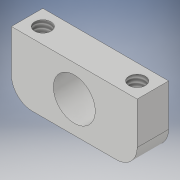
# Autodesk Inventor part: WheelSuspensionHub
Saved by Autodesk Inventor 2017 (Build 210142000, 142)
## iProperties
Created: 2018-05-04
Part Number: WheelSuspensionHub
Material: Generic
Document SubType Name: Modeling
Designer: User
Density: 1 g/cm^3
Appearance: Default
Author: User
Autodesk Inventor part; units mm, degrees
ref_plane "YZ Plane" through (0, 0, 0) normal (1, 0, 0) x (0, 1, 0)
ref_plane "XZ Plane" through (0, 0, 0) normal (0, 1, 0) x (-1, 0, 0)
ref_plane "XY Plane" through (0, 0, 0) normal (0, 0, 1) x (1, 0, 0)
sketch "Sketch1" plane through (0, 0, 0) normal (0, 0, 1) x (1, 0, 0)
  circle A0 centre (0, 0) radius 6.35
  arc A1 (0, 9.525) -> (0, -9.525) centre (0, 0) ccw
  line L0 (0, -9.525) -> (19.05, -9.525)
  line L1 (19.05, -9.525) -> (19.05, 9.525)
  line L2 (19.05, 9.525) -> (0, 9.525)
  dimension "d0" = 12.7
  dimension "d1" = 19.05
  dimension "d2" = 19.05
  dimension "d3" = 19.05
  constraints: 6 end point, 2 centre point, 2 coincident, 2 point on circle, 2 tangent, 1 horizontal, 1 vertical
  measures "d0" diameter of A0
  measures "d1" diameter of A1
  measures "d2" distance of L0.start L0.end
  measures "d3" distance of L0.end L1.end
extrude "Extrusion1" add sketch "Sketch1" along normal blind 9.525
fillet "Fillet1" radius 6.35 1 edges at (19.05, -9.525, 4.7625)
sketch "Sketch2" plane through (0, 9.525, 0) normal (0, 1, 0) x (1, 0, 0)
  line L0 (0, 0) -> (19.05, 0) projected
  line L1 (0, 0) -> (0, -9.525) projected
  line L2 (19.05, -9.525) -> (0, -9.525) projected
  line L3 (19.05, 0) -> (19.05, -9.525) projected
  line L4 (6.35, 0) -> (6.35, -9.525) projected
  point P0 (0, 0)
  point P1 (14.2875, -4.7625)
  dimension "d7" = 4.7625
  dimension "d9" = 9.525
  dimension "d17" = 7.9375
  measures "d7" distance from line of L0 point (14.287, -4.763)
  measures "d9" distance of L0.end L2.start
  measures "d17" distance from line of point (14.287, -4.763) L4
hole "Hole1" at (14.2875, 9.525, 4.7625) direction (0, -1, 0) diameter 4.9784 depth 11.1125 tip angle 118 thread size "1/4-20 UNC" class "2B" standard "ANSI Unified Screw Threads"
mirror "Mirror1" about plane through (0, 0, 0) normal (1, 0, 0) of "Extrusion1", "Hole1", "Fillet1"
equation "\"d7\" = 0.5 * d9"
body "Solid1"
